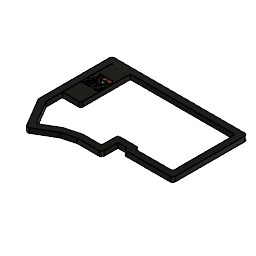
Right_top_cover (Autodesk Fusion 360 design; units mm, degrees)
part number: 2026-07-18-15-23-12-315
Autodesk Fusion 360 part; units mm, degrees
(part 1 of 2)
sketch "Right_enclosure_outline" plane through (0, 0, 0) normal (0, 0, 1) x (1, 0, 0)
  arc A0 (22.5, -32.5) -> (24.5, -34.5) centre (22.5, -34.5) cw
  line L0 (65.0462, 36) -> (-72.8538, 36)
  line L1 (0.5, -49.2983) -> (0.5, -34.5)
  line L2 (67.0462, -34.0424) -> (67.0462, 34)
  line L3 (-21.4538, -51.2983) -> (-1.5, -51.2983)
  line L4 (44.5449, -36.0424) -> (65.0462, -36.0424)
  line L5 (-39.1, -56.2) -> (-21.4538, -51.2983)
  line L6 (24.5, -34.5) -> (24.5, -36.0424)
  line L7 (2.5, -32.5) -> (22.5, -32.5)
  line L8 (-74.8538, 34) -> (-74.8538, 31.6376)
  arc A1 (0.5, -34.5) -> (2.5, -32.5) centre (2.5, -34.5) cw
  line L9 (-74.8538, 0.3904) -> (-74.8538, -39.752)
  line L10 (24.5, -36.0424) -> (44.5449, -36.0424)
  line L11 (-74.8538, 31.6376) -> (-74.8538, 0.3904)
  line L12 (-56.6719, -66.5254) -> (-39.1, -56.2)
  line L13 (-21.4538, -51.2983) -> (-1.5, -51.2983)
  line L14 (2.5, -32.5) -> (22.5, -32.5)
  line L15 (0.5, -49.2983) -> (0.5, -34.5)
  line L16 (24.5, -36.0424) -> (44.5449, -36.0424)
  arc A2 (-72.8538, 36) -> (-74.8538, 34) centre (-72.8538, 34) ccw
  line L17 (44.5449, -36.0424) -> (65.0462, -36.0424)
  line L18 (-74.8538, 0.3904) -> (-74.8538, -39.752)
  line L19 (67.0462, -34.0424) -> (67.0462, 34)
  line L20 (-74.8538, -39.752) -> (-59.4057, -65.8207)
  arc A3 (65.0462, -36.0424) -> (67.0462, -34.0424) centre (65.0462, -34.0424) ccw
  line L21 (-39.1, -56.2) -> (-21.4538, -51.2983)
  arc A4 (67.0462, 34) -> (65.0462, 36) centre (65.0462, 34) ccw
  arc A5 (-59.4057, -65.8207) -> (-56.6719, -66.5254) centre (-57.6851, -64.8011) ccw
  line L22 (24.5, -34.5) -> (24.5, -36.0424)
  arc A6 (-1.5, -51.2983) -> (0.5, -49.2983) centre (-1.5, -49.2983) ccw
  line L23 (-81.8538, 31.6376) -> (-81.8538, 0.3904)
  line L24 (-81.8538, 0.3904) -> (-81.8538, -41.6703)
  line L25 (-81.8538, -41.6703) -> (-62.3802, -74.532)
  line L26 (-58.2795, -75.5891) -> (-36.3436, -62.6994)
  arc A7 (17.5, -40.0424) -> (20.5, -43.0424) centre (20.5, -40.0424) ccw
  line L27 (-36.3436, -62.6994) -> (-20.4997, -58.2983)
  line L28 (71.0462, 43) -> (-78.8538, 43)
  line L29 (7.5, -55.2983) -> (7.5, -39.5)
  line L30 (20.5, -43.0424) -> (44.5449, -43.0424)
  line L31 (44.5449, -43.0424) -> (71.0462, -43.0424)
  line L32 (17.5, -39.5) -> (17.5, -40.0424)
  arc A8 (4.5, -58.2983) -> (7.5, -55.2983) centre (4.5, -55.2983) ccw
  line L33 (-81.8538, 40) -> (-81.8538, 31.6376)
  arc A9 (-62.3802, -74.532) -> (-58.2795, -75.5891) centre (-59.7994, -73.0026) ccw
  arc A10 (74.0462, 40) -> (71.0462, 43) centre (71.0462, 40) ccw
  arc A11 (-78.8538, 43) -> (-81.8538, 40) centre (-78.8538, 40) ccw
  line L34 (-20.4997, -58.2983) -> (4.5, -58.2983)
  line L35 (74.0462, -40.0424) -> (74.0462, 40)
  line L36 (7.5, -39.5) -> (17.5, -39.5)
  arc A12 (71.0462, -43.0424) -> (74.0462, -40.0424) centre (71.0462, -40.0424) ccw
  circle A13 centre (-78, 39) radius 1.6
  circle A14 centre (-60, -71) radius 1.6
  circle A15 centre (69.7169, -39.1925) radius 1.6
  circle A16 centre (69.6831, 39.8042) radius 1.6
  arc A17 (-1.5, -51.2983) -> (0.5, -49.2983) centre (-1.5, -49.2983) ccw
  arc A18 (2.5, -32.5) -> (0.5, -34.5) centre (2.5, -34.5) ccw
  arc A19 (24.5, -34.5) -> (22.5, -32.5) centre (22.5, -34.5) ccw
  arc A20 (65.0462, -36.0424) -> (67.0462, -34.0424) centre (65.0462, -34.0424) ccw
  arc A21 (67.0462, 34) -> (65.0462, 36) centre (65.0462, 34) ccw
  line L37 (-72.8247, 36.0109) -> (-54.3307, 36.0109)
  arc A22 (-72.8247, 36.0109) -> (-74.8247, 34.0109) centre (-72.8247, 34.0109) ccw
  line L38 (-72.8247, 36.0109) -> (-53.7017, 36.0109)
  line L39 (-53.7017, 36.0109) -> (-53.7017, -19.0891)
  line L40 (-55.7017, -21.0891) -> (-74.8247, -21.0891)
  line L41 (-74.8247, -21.0891) -> (-74.8247, 34.0109)
  arc A23 (-72.8247, 36.0109) -> (-74.8247, 34.0109) centre (-72.8247, 34.0109) ccw
  arc A24 (-55.7017, -21.0891) -> (-53.7017, -19.0891) centre (-55.7017, -19.0891) ccw
  point P0 (-74.8247, 36.0109)
  point P1 (-74.8247, 36.0109)
  dimension "d4" = 20.494
  dimension "d6" = 2
  dimension "d8" = 57.1
  dimension "d9" = 2
  constraint tangent L1 A17
  constraint tangent L3 A17
  constraint tangent L14 A18
  constraint tangent L15 A18
  constraint tangent L14 A19
  constraint tangent L22 A19
  constraint tangent L2 A20
  constraint tangent L4 A20
  constraint tangent L0 A21
  constraint tangent L2 A21
  constraint horizontal L37
  constraint coincident P1 L37
  constraint tangent L37 A22
  constraint perpendicular L38 L39
  constraint parallel L38 L40
  constraint parallel L39 L41
  constraint parallel L0 L38
  constraint coincident P1 P0
  constraint coincident P1 L38
  constraint coincident P1 L41
  constraint tangent L38 A23
  constraint tangent L41 A23
  constraint tangent L39 A24
  constraint tangent L40 A24
  constraint equal A23 A24
  measures "d4" distance of P1 L37.end
  measures "d6" radius of A22
  measures "d8" distance of P1 L40.end
  measures "d9" radius of A23
extrude "Extrude1" add sketch "Right_enclosure_outline" along normal blind 4.5 contours L0 A2 L37 A22 L38 L39 A23 | L23 L24 L25 L26 A7 L27 L28 L29 L30 L31 L32 A8 L33 A9 A10 A11 L34 L35 L36 A12 | A13 | A14 | A15 | A16 makes body 1
extrude "Extrude2" add sketch "Right_enclosure_outline" along normal blind 4.5 contours L0 A2 A22 L39 L40 L41 A23 A24 bodies 1
extrude "Extrude3" add 1 faces at (-67.7837, -2.0557, 4.5) along direction (0, 0, 1) blind 0.5 on bodies 1 bodies 1
extrude "Extrude4" add 1 faces at (-67.7837, -2.0557, 5) along direction (0, 0, 1) blind 0.5 on bodies 1 bodies 1
sketch "Sketch2" plane through (0, 0, 0) normal (0, 0, 1) x (1, 0, 0)
  circle A0 centre (-60, -71) radius 1.6
  circle A1 centre (-78, 39) radius 1.6
  circle A2 centre (69.6831, 39.8042) radius 1.6
  circle A3 centre (69.7169, -39.1925) radius 1.6
  circle A4 centre (-60, -71) radius 2.45
  circle A5 centre (-78, 39) radius 2.45
  circle A6 centre (69.6831, 39.8042) radius 2.45
  circle A7 centre (69.7169, -39.1925) radius 2.45
  dimension "d16" = 4.9
  dimension "d17" = 4.9
  dimension "d18" = 4.9
  dimension "d19" = 4.9
  constraint concentric A0 A4
  constraint concentric A1 A5
  constraint concentric A2 A6
  constraint concentric A3 A7
  measures "d16" diameter of A4
  measures "d17" diameter of A5
  measures "d18" diameter of A6
  measures "d19" diameter of A7
extrude "Extrude5" cut sketch "Sketch2" along normal blind 3.9 contours A0 | A1 | A2 | A3 | A4 | A5 | A6 | A7 bodies 1
sketch "Sketch3" plane through (0, 0, 0) normal (0, 0, -1) x (1, 0, 0)
  arc A0 (74.0462, 40.0424) -> (71.0462, 43.0424) centre (71.0462, 40.0424) ccw
  line L0 (71.0462, 43.0424) -> (20.5, 43.0424)
  arc A1 (20.5, 43.0424) -> (17.5, 40.0424) centre (20.5, 40.0424) ccw
  line L1 (17.5, 40.0424) -> (17.5, 39.5)
  line L2 (17.5, 39.5) -> (7.5, 39.5)
  line L3 (7.5, 39.5) -> (7.5, 55.2983)
  arc A2 (7.5, 55.2983) -> (4.5, 58.2983) centre (4.5, 55.2983) ccw
  line L4 (4.5, 58.2983) -> (-20.4997, 58.2983)
  line L5 (-20.4997, 58.2983) -> (-36.3436, 62.6994)
  line L6 (-36.3436, 62.6994) -> (-58.2795, 75.5891)
  arc A3 (-58.2795, 75.5891) -> (-62.3802, 74.532) centre (-59.7994, 73.0026) ccw
  line L7 (-62.3802, 74.532) -> (-81.8538, 41.6703)
  line L8 (-81.8538, 41.6703) -> (-81.8538, -40)
  arc A4 (-81.8538, -40) -> (-78.8538, -43) centre (-78.8538, -40) ccw
  line L9 (-78.8538, -43) -> (71.0462, -43)
  arc A5 (71.0462, -43) -> (74.0462, -40) centre (71.0462, -40) ccw
  line L10 (74.0462, -40) -> (74.0462, 40.0424)
  line L11 (24.5, 34.5) -> (24.5, 36.0424)
  line L12 (24.5, 36.0424) -> (65.0462, 36.0424)
  arc A6 (67.0462, 34.0424) -> (65.0462, 36.0424) centre (65.0462, 34.0424) ccw
  line L13 (67.0462, 34.0424) -> (67.0462, -34)
  arc A7 (65.0462, -36) -> (67.0462, -34) centre (65.0462, -34) ccw
  line L14 (65.0462, -36) -> (-53.7017, -36)
  line L15 (-53.7017, -36) -> (-53.7017, 19.0891)
  arc A8 (-53.7017, 19.0891) -> (-55.7017, 21.0891) centre (-55.7017, 19.0891) ccw
  line L16 (-55.7017, 21.0891) -> (-74.8247, 21.0891)
  line L17 (-74.8247, 21.0891) -> (-74.8247, -34.0109)
  arc A9 (-74.8247, -34.0109) -> (-73.5427, -35.8776) centre (-72.8247, -34.0109) ccw
  arc A10 (-74.8538, -34) -> (-73.5427, -35.8776) centre (-72.8538, -34) ccw
  line L18 (-74.8538, -34) -> (-74.8538, 39.752)
  line L19 (-74.8538, 39.752) -> (-59.4057, 65.8207)
  arc A11 (-56.6719, 66.5254) -> (-59.4057, 65.8207) centre (-57.6851, 64.8011) ccw
  line L20 (-56.6719, 66.5254) -> (-39.1, 56.2)
  line L21 (-39.1, 56.2) -> (-21.4538, 51.2983)
  line L22 (-21.4538, 51.2983) -> (-1.5, 51.2983)
  arc A12 (0.5, 49.2983) -> (-1.5, 51.2983) centre (-1.5, 49.2983) ccw
  line L23 (0.5, 49.2983) -> (0.5, 34.5)
  arc A13 (0.5, 34.5) -> (2.5, 32.5) centre (2.5, 34.5) ccw
  line L24 (2.5, 32.5) -> (22.5, 32.5)
  arc A14 (22.5, 32.5) -> (24.5, 34.5) centre (22.5, 34.5) ccw
  circle A15 centre (69.7169, 39.1925) radius 2.45
  circle A16 centre (-60, 71) radius 2.45
  circle A17 centre (69.6831, -39.8042) radius 2.45
  circle A18 centre (-78, -39) radius 2.45
  line L25 (-74, 19) -> (-55, 19)
  line L26 (-55, 19) -> (-55, -33)
  line L27 (-55, -33) -> (-74, -33)
  line L28 (-74, -33) -> (-74, 19)
  constraint perpendicular L25 L26
  constraint parallel L25 L27
  constraint parallel L26 L28
  constraint perpendicular L15 L25
extrude "Extrude6" cut sketch "Sketch3" against normal blind 4.5 contours L25 L26 L27 L28 bodies 1
sketch "Sketch4" plane through (0, 0, 5.5) normal (0, 0, 1) x (-1, 0, 0)
  line L0 (-24.5, 36.0424) -> (-24.5, 34.5)
  arc A0 (-24.5, 34.5) -> (-22.5, 32.5) centre (-22.5, 34.5) ccw
  line L1 (-22.5, 32.5) -> (-2.5, 32.5)
  arc A1 (-2.5, 32.5) -> (-0.5, 34.5) centre (-2.5, 34.5) ccw
  line L2 (-0.5, 34.5) -> (-0.5, 49.2983)
  arc A2 (1.5, 51.2983) -> (-0.5, 49.2983) centre (1.5, 49.2983) ccw
  line L3 (1.5, 51.2983) -> (21.4538, 51.2983)
  line L4 (21.4538, 51.2983) -> (39.1, 56.2)
  line L5 (39.1, 56.2) -> (56.6719, 66.5254)
  arc A3 (59.4057, 65.8207) -> (56.6719, 66.5254) centre (57.6851, 64.8011) ccw
  line L6 (59.4057, 65.8207) -> (74.8538, 39.752)
  line L7 (74.8538, 39.752) -> (74.8538, -34)
  arc A4 (73.5427, -35.8776) -> (74.8538, -34) centre (72.8538, -34) ccw
  arc A5 (73.5427, -35.8776) -> (74.8247, -34.0109) centre (72.8247, -34.0109) ccw
  line L8 (74.8247, -34.0109) -> (74.8247, 21.0891)
  line L9 (74.8247, 21.0891) -> (55.7017, 21.0891)
  arc A6 (55.7017, 21.0891) -> (53.7017, 19.0891) centre (55.7017, 19.0891) ccw
  line L10 (53.7017, 19.0891) -> (53.7017, -36)
  line L11 (53.7017, -36) -> (-65.0462, -36)
  arc A7 (-67.0462, -34) -> (-65.0462, -36) centre (-65.0462, -34) ccw
  line L12 (-67.0462, -34) -> (-67.0462, 34.0424)
  arc A8 (-65.0462, 36.0424) -> (-67.0462, 34.0424) centre (-65.0462, 34.0424) ccw
  line L13 (-65.0462, 36.0424) -> (-24.5, 36.0424)
  arc A9 (-71.0462, 43.0424) -> (-74.0462, 40.0424) centre (-71.0462, 40.0424) ccw
  line L14 (-74.0462, 40.0424) -> (-74.0462, -40)
  arc A10 (-74.0462, -40) -> (-71.0462, -43) centre (-71.0462, -40) ccw
  line L15 (-71.0462, -43) -> (78.8538, -43)
  arc A11 (78.8538, -43) -> (81.8538, -40) centre (78.8538, -40) ccw
  line L16 (81.8538, -40) -> (81.8538, 41.6703)
  line L17 (81.8538, 41.6703) -> (62.3802, 74.532)
  arc A12 (62.3802, 74.532) -> (58.2795, 75.5891) centre (59.7994, 73.0026) ccw
  line L18 (58.2795, 75.5891) -> (36.3436, 62.6994)
  line L19 (36.3436, 62.6994) -> (20.4997, 58.2983)
  line L20 (20.4997, 58.2983) -> (-4.5, 58.2983)
  arc A13 (-4.5, 58.2983) -> (-7.5, 55.2983) centre (-4.5, 55.2983) ccw
  line L21 (-7.5, 55.2983) -> (-7.5, 39.5)
  line L22 (-7.5, 39.5) -> (-17.5, 39.5)
  line L23 (-17.5, 39.5) -> (-17.5, 40.0424)
  arc A14 (-17.5, 40.0424) -> (-20.5, 43.0424) centre (-20.5, 40.0424) ccw
  line L24 (-20.5, 43.0424) -> (-71.0462, 43.0424)
  spline S0 degree 3 poles (70.819, -18.6802) (70.9391, -18.6554) (71.1029, -18.5716) (71.16, -18.503) knots 0 0 0 0 1 1 1 1
  spline S1 degree 3 poles (71.16, -18.503) (71.2553, -18.3906) (71.2896, -18.2859) (71.2896, -18.1087) knots 0 0 0 0 1 1 1 1
  spline S2 degree 3 poles (71.2896, -18.1087) (71.2877, -17.9106) (71.2439, -17.8039) (71.1105, -17.6839) knots 0 0 0 0 1 1 1 1
  spline S3 degree 3 poles (71.1105, -17.6839) (70.9486, -17.5391) (70.7562, -17.5086) (70.379, -17.5677) knots 0 0 0 0 1 1 1 1
  spline S4 degree 3 poles (70.379, -17.5677) (70.1466, -17.6058) (69.9866, -17.5963) (69.9142, -17.5448) knots 0 0 0 0 1 1 1 1
  spline S5 degree 3 poles (69.9142, -17.5448) (69.8399, -17.4896) (69.7465, -17.3429) (69.718, -17.2381) knots 0 0 0 0 1 1 1 1
  spline S6 degree 3 poles (69.718, -17.2381) (69.6856, -17.1181) (69.6703, -11.8108) (69.7008, -11.6031) knots 0 0 0 0 1 1 1 1
  spline S7 degree 3 poles (69.7008, -11.6031) (69.7122, -11.5307) (69.7465, -11.4164) (69.7789, -11.3517) knots 0 0 0 0 1 1 1 1
  spline S8 degree 3 poles (69.7789, -11.3517) (69.8246, -11.2564) (69.8551, -11.2221) (69.9256, -11.1802) knots 0 0 0 0 1 1 1 1
  spline S9 degree 3 poles (69.9256, -11.1802) (70.0285, -11.1193) (70.1256, -11.1155) (70.4819, -11.1536) knots 0 0 0 0 1 1 1 1
  spline S10 degree 3 poles (70.4819, -11.1536) (70.9372, -11.2031) (71.1315, -11.1345) (71.2458, -10.8792) knots 0 0 0 0 1 1 1 1
  spline S11 degree 3 poles (71.2458, -10.8792) (71.2801, -10.8049) (71.2896, -10.7478) (71.2896, -10.6202) knots 0 0 0 0 1 1 1 1
  spline S12 degree 3 poles (71.2896, -10.6202) (71.2896, -10.4716) (71.2839, -10.4449) (71.2248, -10.3249) knots 0 0 0 0 1 1 1 1
  spline S13 degree 3 poles (71.2248, -10.3249) (71.0705, -10.0201) (70.7733, -9.9534) (70.0628, -10.0677) knots 0 0 0 0 1 1 1 1
  spline S14 degree 3 poles (70.0628, -10.0677) (69.5675, -10.1458) (69.2855, -10.1687) (68.8626, -10.1687) knots 0 0 0 0 1 1 1 1
  spline S15 degree 3 poles (68.8626, -10.1687) (68.5083, -10.1668) (68.4454, -10.161) (67.7577, -10.0506) knots 0 0 0 0 1 1 1 1
  spline S16 degree 3 poles (67.7577, -10.0506) (67.3558, -9.9877) (67.0929, -10.0067) (66.8967, -10.1172) knots 0 0 0 0 1 1 1 1
  spline S17 degree 3 poles (66.8967, -10.1172) (66.7233, -10.2144) (66.6547, -10.3401) (66.6395, -10.584) knots 0 0 0 0 1 1 1 1
  spline S18 degree 3 poles (66.6395, -10.584) (66.6242, -10.8526) (66.7138, -11.0297) (66.9195, -11.125) knots 0 0 0 0 1 1 1 1
  spline S19 degree 3 poles (66.9195, -11.125) (66.99, -11.1574) (67.0414, -11.165) (67.2148, -11.165) knots 0 0 0 0 1 1 1 1
  spline S20 degree 3 poles (67.2148, -11.165) (67.3291, -11.165) (67.5158, -11.1536) (67.6282, -11.1402) knots 0 0 0 0 1 1 1 1
  spline S21 degree 3 poles (67.6282, -11.1402) (67.8796, -11.1097) (67.9635, -11.1269) (68.0644, -11.2278) knots 0 0 0 0 1 1 1 1
  spline S22 degree 3 poles (68.0644, -11.2278) (68.1025, -11.2679) (68.154, -11.3498) (68.1787, -11.4126) knots 0 0 0 0 1 1 1 1
  line L25 (68.1787, -11.4126) -> (68.2244, -11.5269)
  line L26 (68.2244, -11.5269) -> (68.2244, -14.3463)
  spline S23 degree 3 poles (68.2244, -14.3463) (68.2244, -17.0267) (68.2225, -17.1714) (68.1901, -17.2743) knots 0 0 0 0 1 1 1 1
  spline S24 degree 3 poles (68.1901, -17.2743) (68.0949, -17.5696) (67.9501, -17.6363) (67.5482, -17.5658) knots 0 0 0 0 1 1 1 1
  spline S25 degree 3 poles (67.5482, -17.5658) (67.1786, -17.501) (66.969, -17.5429) (66.7957, -17.7163) knots 0 0 0 0 1 1 1 1
  spline S26 degree 3 poles (66.7957, -17.7163) (66.6814, -17.8287) (66.6338, -17.9468) (66.6338, -18.1106) knots 0 0 0 0 1 1 1 1
  spline S27 degree 3 poles (66.6338, -18.1106) (66.6338, -18.2744) (66.6852, -18.4078) (66.7862, -18.5107) knots 0 0 0 0 1 1 1 1
  spline S28 degree 3 poles (66.7862, -18.5107) (66.9805, -18.7069) (67.2567, -18.7393) (67.9101, -18.644) knots 0 0 0 0 1 1 1 1
  spline S29 degree 3 poles (67.9101, -18.644) (68.7655, -18.5221) (69.1807, -18.5221) (70.0056, -18.6421) knots 0 0 0 0 1 1 1 1
  spline S30 degree 3 poles (70.0056, -18.6421) (70.3942, -18.6993) (70.659, -18.7107) (70.819, -18.6802) knots 0 0 0 0 1 1 1 1
  spline S31 degree 3 poles (63.0143, -18.5926) (63.3648, -18.5392) (63.7648, -18.404) (64.062, -18.2382) knots 0 0 0 0 1 1 1 1
  spline S32 degree 3 poles (64.062, -18.2382) (64.2582, -18.1297) (64.5592, -17.8953) (64.6983, -17.7449) knots 0 0 0 0 1 1 1 1
  spline S33 degree 3 poles (64.6983, -17.7449) (65.045, -17.3696) (65.3612, -16.7123) (65.445, -16.1923) knots 0 0 0 0 1 1 1 1
  spline S34 degree 3 poles (65.445, -16.1923) (65.5098, -15.7922) (65.4984, -15.0055) (65.426, -14.7026) knots 0 0 0 0 1 1 1 1
  spline S35 degree 3 poles (65.426, -14.7026) (65.3326, -14.3159) (65.1155, -13.7939) (64.8774, -13.3748) knots 0 0 0 0 1 1 1 1
  spline S36 degree 3 poles (64.8774, -13.3748) (64.5802, -12.8566) (64.1268, -12.2718) (63.6448, -11.7879) knots 0 0 0 0 1 1 1 1
  spline S37 degree 3 poles (63.6448, -11.7879) (62.9343, -11.0735) (62.0884, -10.4506) (60.9664, -9.8181) knots 0 0 0 0 1 1 1 1
  spline S38 degree 3 poles (60.9664, -9.8181) (60.8826, -9.7705) (60.7797, -9.7115) (60.7378, -9.6886) knots 0 0 0 0 1 1 1 1
  spline S39 degree 3 poles (60.7378, -9.6886) (60.5911, -9.6048) (60.3663, -9.4981) (60.3377, -9.4981) knots 0 0 0 0 1 1 1 1
  spline S40 degree 3 poles (60.3377, -9.4981) (60.2577, -9.4981) (59.791, -9.7762) (59.0614, -10.2601) knots 0 0 0 0 1 1 1 1
  spline S41 degree 3 poles (59.0614, -10.2601) (58.6556, -10.5287) (58.2289, -10.843) (57.9851, -11.0507) knots 0 0 0 0 1 1 1 1
  spline S42 degree 3 poles (57.9851, -11.0507) (57.9584, -11.0735) (57.8689, -11.1516) (57.785, -11.224) knots 0 0 0 0 1 1 1 1
  spline S43 degree 3 poles (57.785, -11.224) (57.1011, -11.8089) (56.282, -12.7252) (55.9086, -13.3253) knots 0 0 0 0 1 1 1 1
  spline S44 degree 3 poles (55.9086, -13.3253) (55.3562, -14.2149) (55.1371, -15.3331) (55.3295, -16.2799) knots 0 0 0 0 1 1 1 1
  spline S45 degree 3 poles (55.3295, -16.2799) (55.4628, -16.9276) (55.8858, -17.6248) (56.3715, -18.0001) knots 0 0 0 0 1 1 1 1
  spline S46 degree 3 poles (56.3715, -18.0001) (57.0173, -18.4992) (57.8631, -18.705) (58.6232, -18.5488) knots 0 0 0 0 1 1 1 1
  spline S47 degree 3 poles (58.6232, -18.5488) (58.9185, -18.4878) (59.1452, -18.383) (59.5186, -18.1354) knots 0 0 0 0 1 1 1 1
  spline S48 degree 3 poles (59.5186, -18.1354) (59.8081, -17.943) (59.9586, -17.8191) (60.2177, -17.5639) knots 0 0 0 0 1 1 1 1
  spline S49 degree 3 poles (60.2177, -17.5639) (60.3396, -17.442) (60.452, -17.3467) (60.4654, -17.3505) knots 0 0 0 0 1 1 1 1
  spline S50 degree 3 poles (60.4654, -17.3505) (60.4806, -17.3524) (60.5568, -17.4286) (60.6349, -17.5182) knots 0 0 0 0 1 1 1 1
  spline S51 degree 3 poles (60.6349, -17.5182) (60.854, -17.7715) (61.1455, -18.0497) (61.3131, -18.1716) knots 0 0 0 0 1 1 1 1
  spline S52 degree 3 poles (61.3131, -18.1716) (61.8389, -18.5469) (62.3951, -18.684) (63.0143, -18.5926) knots 0 0 0 0 1 1 1 1
  spline S53 degree 3 poles (60.7206, -16.0018) (60.7016, -15.9942) (60.6902, -15.9675) (60.6902, -15.9275) knots 0 0 0 0 1 1 1 1
  spline S54 degree 3 poles (60.6902, -15.9275) (60.6902, -15.8913) (60.6806, -15.857) (60.6711, -15.8513) knots 0 0 0 0 1 1 1 1
  spline S55 degree 3 poles (60.6711, -15.8513) (60.6463, -15.836) (60.6463, -15.7275) (60.6711, -15.7275) knots 0 0 0 0 1 1 1 1
  spline S56 degree 3 poles (60.6711, -15.7275) (60.6959, -15.7275) (60.6806, -15.5732) (60.6387, -15.4093) knots 0 0 0 0 1 1 1 1
  spline S57 degree 3 poles (60.6387, -15.4093) (60.6159, -15.316) (60.6006, -15.2893) (60.574, -15.2893) knots 0 0 0 0 1 1 1 1
  spline S58 degree 3 poles (60.574, -15.2893) (60.532, -15.2893) (60.5282, -15.3103) (60.5606, -15.3426) knots 0 0 0 0 1 1 1 1
  spline S59 degree 3 poles (60.5606, -15.3426) (60.5778, -15.3598) (60.5778, -15.3655) (60.5625, -15.3655) knots 0 0 0 0 1 1 1 1
  spline S60 degree 3 poles (60.5625, -15.3655) (60.5492, -15.3655) (60.534, -15.3579) (60.5282, -15.3465) knots 0 0 0 0 1 1 1 1
  spline S61 degree 3 poles (60.5282, -15.3465) (60.5073, -15.3141) (60.4616, -15.3255) (60.4616, -15.3636) knots 0 0 0 0 1 1 1 1
  spline S62 degree 3 poles (60.4616, -15.3636) (60.4616, -15.4227) (60.4254, -15.4303) (60.4025, -15.3769) knots 0 0 0 0 1 1 1 1
  spline S63 degree 3 poles (60.4025, -15.3769) (60.3835, -15.3388) (60.3739, -15.3331) (60.3377, -15.3465) knots 0 0 0 0 1 1 1 1
  spline S64 degree 3 poles (60.3377, -15.3465) (60.3015, -15.3598) (60.2958, -15.3579) (60.3034, -15.3255) knots 0 0 0 0 1 1 1 1
  spline S65 degree 3 poles (60.3034, -15.3255) (60.3111, -15.3007) (60.3034, -15.2893) (60.2844, -15.2893) knots 0 0 0 0 1 1 1 1
  spline S66 degree 3 poles (60.2844, -15.2893) (60.2615, -15.2893) (60.2558, -15.276) (60.2634, -15.2283) knots 0 0 0 0 1 1 1 1
  spline S67 degree 3 poles (60.2634, -15.2283) (60.2901, -15.0645) (60.2825, -15.0169) (60.2196, -14.9426) knots 0 0 0 0 1 1 1 1
  spline S68 degree 3 poles (60.2196, -14.9426) (60.1872, -14.9026) (60.1549, -14.8454) (60.1472, -14.815) knots 0 0 0 0 1 1 1 1
  spline S69 degree 3 poles (60.1472, -14.815) (60.1415, -14.7845) (60.1225, -14.7483) (60.1053, -14.735) knots 0 0 0 0 1 1 1 1
  spline S70 degree 3 poles (60.1053, -14.735) (60.0825, -14.714) (60.0729, -14.7159) (60.052, -14.7426) knots 0 0 0 0 1 1 1 1
  spline S71 degree 3 poles (60.052, -14.7426) (60.0234, -14.7826) (59.9986, -14.7826) (59.9263, -14.7464) knots 0 0 0 0 1 1 1 1
  spline S72 degree 3 poles (59.9263, -14.7464) (59.8729, -14.7178) (59.871, -14.7102) (59.8767, -14.6264) knots 0 0 0 0 1 1 1 1
  spline S73 degree 3 poles (59.8767, -14.6264) (59.8843, -14.5292) (59.9072, -14.4721) (59.9548, -14.4321) knots 0 0 0 0 1 1 1 1
  spline S74 degree 3 poles (59.9548, -14.4321) (59.972, -14.4187) (59.9853, -14.3825) (59.9853, -14.352) knots 0 0 0 0 1 1 1 1
  spline S75 degree 3 poles (59.9853, -14.352) (59.9853, -14.3178) (60.0025, -14.2797) (60.0329, -14.253) knots 0 0 0 0 1 1 1 1
  spline S76 degree 3 poles (60.0329, -14.253) (60.0748, -14.213) (60.0787, -14.2016) (60.0672, -14.0777) knots 0 0 0 0 1 1 1 1
  spline S77 degree 3 poles (60.0672, -14.0777) (60.0615, -14.0053) (60.0672, -13.8415) (60.0787, -13.712) knots 0 0 0 0 1 1 1 1
  spline S78 degree 3 poles (60.0787, -13.712) (60.1053, -13.4472) (60.0958, -13.3748) (60.0387, -13.3595) knots 0 0 0 0 1 1 1 1
  spline S79 degree 3 poles (60.0387, -13.3595) (60.0082, -13.35) (60.0025, -13.3367) (60.0082, -13.3005) knots 0 0 0 0 1 1 1 1
  spline S80 degree 3 poles (60.0082, -13.3005) (60.0177, -13.2567) (60.012, -13.2529) (59.9301, -13.2471) knots 0 0 0 0 1 1 1 1
  line L27 (59.9301, -13.2471) -> (59.8424, -13.2414)
  line L28 (59.8424, -13.2414) -> (59.8367, -13.1614)
  spline S81 degree 3 poles (59.8367, -13.1614) (59.8329, -13.1119) (59.8386, -13.0795) (59.852, -13.0795) knots 0 0 0 0 1 1 1 1
  spline S82 degree 3 poles (59.852, -13.0795) (59.8824, -13.0795) (59.8691, -12.428) (59.8367, -12.4166) knots 0 0 0 0 1 1 1 1
  spline S83 degree 3 poles (59.8367, -12.4166) (59.8196, -12.4109) (59.8139, -12.4909) (59.8139, -12.7709) knots 0 0 0 0 1 1 1 1
  spline S84 degree 3 poles (59.8139, -12.7709) (59.8139, -13.1176) (59.812, -13.1348) (59.7758, -13.1462) knots 0 0 0 0 1 1 1 1
  spline S85 degree 3 poles (59.7758, -13.1462) (59.7396, -13.1576) (59.7377, -13.1748) (59.7377, -13.6682) knots 0 0 0 0 1 1 1 1
  line L29 (59.7377, -13.6682) -> (59.7377, -14.1787)
  line L30 (59.7377, -14.1787) -> (59.551, -14.192)
  spline S86 degree 3 poles (59.551, -14.192) (59.45, -14.1977) (59.3071, -14.2092) (59.2366, -14.2149) knots 0 0 0 0 1 1 1 1
  spline S87 degree 3 poles (59.2366, -14.2149) (59.1604, -14.2225) (59.0881, -14.2187) (59.0652, -14.2073) knots 0 0 0 0 1 1 1 1
  spline S88 degree 3 poles (59.0652, -14.2073) (59.0423, -14.1958) (59.008, -14.1825) (58.989, -14.1768) knots 0 0 0 0 1 1 1 1
  spline S89 degree 3 poles (58.989, -14.1768) (58.9661, -14.1692) (58.9566, -14.1463) (58.9566, -14.1006) knots 0 0 0 0 1 1 1 1
  spline S90 degree 3 poles (58.9566, -14.1006) (58.9566, -14.0434) (58.9509, -14.0339) (58.9033, -14.0282) knots 0 0 0 0 1 1 1 1
  line L31 (58.9033, -14.0282) -> (58.8518, -14.0225)
  line L32 (58.8518, -14.0225) -> (58.8385, -13.7367)
  spline S91 degree 3 poles (58.8385, -13.7367) (58.8214, -13.3329) (58.808, -13.2567) (58.7642, -13.2452) knots 0 0 0 0 1 1 1 1
  spline S92 degree 3 poles (58.7642, -13.2452) (58.7337, -13.2376) (58.728, -13.2186) (58.728, -13.1367) knots 0 0 0 0 1 1 1 1
  line L33 (58.728, -13.1367) -> (58.728, -13.0376)
  line L34 (58.728, -13.0376) -> (58.6709, -13.0509)
  spline S93 degree 3 poles (58.6709, -13.0509) (58.6385, -13.0586) (58.5661, -13.0643) (58.5089, -13.0643) knots 0 0 0 0 1 1 1 1
  line L35 (58.5089, -13.0643) -> (58.4042, -13.0662)
  line L36 (58.4042, -13.0662) -> (58.4042, -13.6243)
  line L37 (58.4042, -13.6243) -> (58.4042, -14.1844)
  line L38 (58.4042, -14.1844) -> (58.3032, -14.1863)
  spline S94 degree 3 poles (58.3032, -14.1863) (58.2499, -14.1863) (58.1089, -14.1882) (57.9908, -14.1882) knots 0 0 0 0 1 1 1 1
  line L39 (57.9908, -14.1882) -> (57.7774, -14.1901)
  line L40 (57.7774, -14.1901) -> (57.7717, -14.2397)
  spline S95 degree 3 poles (57.7717, -14.2397) (57.7679, -14.2682) (57.7546, -14.2892) (57.7374, -14.2892) knots 0 0 0 0 1 1 1 1
  spline S96 degree 3 poles (57.7374, -14.2892) (57.7165, -14.2892) (57.7069, -14.2587) (57.6974, -14.1749) knots 0 0 0 0 1 1 1 1
  spline S97 degree 3 poles (57.6974, -14.1749) (57.6917, -14.112) (57.6669, -14.0053) (57.6422, -13.9368) knots 0 0 0 0 1 1 1 1
  spline S98 degree 3 poles (57.6422, -13.9368) (57.6174, -13.8682) (57.5926, -13.7463) (57.5869, -13.6605) knots 0 0 0 0 1 1 1 1
  line L41 (57.5869, -13.6605) -> (57.5755, -13.5081)
  line L42 (57.5755, -13.5081) -> (57.4707, -13.5024)
  spline S99 degree 3 poles (57.4707, -13.5024) (57.4136, -13.4986) (57.3602, -13.4853) (57.3526, -13.4738) knots 0 0 0 0 1 1 1 1
  spline S100 degree 3 poles (57.3526, -13.4738) (57.345, -13.4605) (57.3374, -13.3195) (57.3374, -13.1576) knots 0 0 0 0 1 1 1 1
  spline S101 degree 3 poles (57.3374, -13.1576) (57.3374, -12.9004) (57.3336, -12.8681) (57.3069, -12.8776) knots 0 0 0 0 1 1 1 1
  spline S102 degree 3 poles (57.3069, -12.8776) (57.2897, -12.8833) (57.2516, -12.889) (57.2231, -12.889) knots 0 0 0 0 1 1 1 1
  spline S103 degree 3 poles (57.2231, -12.889) (57.1716, -12.889) (57.1678, -12.8947) (57.1621, -12.9709) knots 0 0 0 0 1 1 1 1
  line L43 (57.1621, -12.9709) -> (57.1564, -13.0509)
  line L44 (57.1564, -13.0509) -> (56.9887, -13.0509)
  line L45 (56.9887, -13.0509) -> (56.823, -13.0509)
  line L46 (56.823, -13.0509) -> (56.823, -13.4186)
  spline S104 degree 3 poles (56.823, -13.4186) (56.823, -13.6434) (56.8154, -13.8015) (56.8021, -13.8244) knots 0 0 0 0 1 1 1 1
  spline S105 degree 3 poles (56.8021, -13.8244) (56.7906, -13.8453) (56.724, -13.9006) (56.6535, -13.9463) knots 0 0 0 0 1 1 1 1
  spline S106 degree 3 poles (56.6535, -13.9463) (56.5373, -14.0206) (56.522, -14.0396) (56.4934, -14.1292) knots 0 0 0 0 1 1 1 1
  spline S107 degree 3 poles (56.4934, -14.1292) (56.4763, -14.1825) (56.4592, -14.2492) (56.4592, -14.2778) knots 0 0 0 0 1 1 1 1
  spline S108 degree 3 poles (56.4592, -14.2778) (56.4573, -14.3082) (56.4496, -14.2911) (56.4344, -14.2282) knots 0 0 0 0 1 1 1 1
  spline S109 degree 3 poles (56.4344, -14.2282) (56.423, -14.1749) (56.4077, -14.1234) (56.3982, -14.1158) knots 0 0 0 0 1 1 1 1
  spline S110 degree 3 poles (56.3982, -14.1158) (56.3906, -14.1082) (56.3849, -14.0777) (56.3849, -14.0492) knots 0 0 0 0 1 1 1 1
  spline S111 degree 3 poles (56.3849, -14.0492) (56.3849, -14.0206) (56.3772, -13.992) (56.3677, -13.9863) knots 0 0 0 0 1 1 1 1
  spline S112 degree 3 poles (56.3677, -13.9863) (56.3468, -13.973) (56.3277, -13.8587) (56.3163, -13.6662) knots 0 0 0 0 1 1 1 1
  spline S113 degree 3 poles (56.3163, -13.6662) (56.3087, -13.55) (56.2991, -13.5177) (56.2763, -13.5177) knots 0 0 0 0 1 1 1 1
  spline S114 degree 3 poles (56.2763, -13.5177) (56.261, -13.5177) (56.2439, -13.5005) (56.2382, -13.4796) knots 0 0 0 0 1 1 1 1
  spline S115 degree 3 poles (56.2382, -13.4796) (56.2325, -13.4586) (56.2153, -13.4415) (56.202, -13.4415) knots 0 0 0 0 1 1 1 1
  spline S116 degree 3 poles (56.202, -13.4415) (56.1601, -13.4415) (56.1696, -13.4129) (56.2629, -13.2757) knots 0 0 0 0 1 1 1 1
  spline S117 degree 3 poles (56.2629, -13.2757) (56.4934, -12.9404) (56.9316, -12.4242) (57.3393, -12.0127) knots 0 0 0 0 1 1 1 1
  spline S118 degree 3 poles (57.3393, -12.0127) (58.0384, -11.306) (58.6823, -10.8049) (59.7472, -10.1325) knots 0 0 0 0 1 1 1 1
  spline S119 degree 3 poles (59.7472, -10.1325) (59.9758, -9.9877) (60.2768, -9.8105) (60.3168, -9.7972) knots 0 0 0 0 1 1 1 1
  spline S120 degree 3 poles (60.3168, -9.7972) (60.353, -9.782) (60.5111, -9.862) (60.8673, -10.0734) knots 0 0 0 0 1 1 1 1
  spline S121 degree 3 poles (60.8673, -10.0734) (60.9721, -10.1344) (61.0578, -10.1839) (61.0616, -10.1839) knots 0 0 0 0 1 1 1 1
  spline S122 degree 3 poles (61.0616, -10.1839) (61.0788, -10.1839) (61.6446, -10.5344) (61.8617, -10.6792) knots 0 0 0 0 1 1 1 1
  spline S123 degree 3 poles (61.8617, -10.6792) (62.9952, -11.4336) (63.9306, -12.3537) (64.5192, -13.2929) knots 0 0 0 0 1 1 1 1
  spline S124 degree 3 poles (64.5192, -13.2929) (64.563, -13.3653) (64.5954, -13.4319) (64.5916, -13.4453) knots 0 0 0 0 1 1 1 1
  spline S125 degree 3 poles (64.5916, -13.4453) (64.5859, -13.4605) (64.5535, -13.4662) (64.504, -13.4643) knots 0 0 0 0 1 1 1 1
  line L47 (64.504, -13.4643) -> (64.4259, -13.4586)
  line L48 (64.4259, -13.4586) -> (64.4202, -13.7024)
  line L49 (64.4202, -13.7024) -> (64.4144, -13.9463)
  line L50 (64.4144, -13.9463) -> (64.2239, -13.9463)
  line L51 (64.2239, -13.9463) -> (64.0334, -13.9463)
  line L52 (64.0334, -13.9463) -> (64.0277, -13.7615)
  line L53 (64.0277, -13.7615) -> (64.022, -13.5748)
  line L54 (64.022, -13.5748) -> (63.8429, -13.5748)
  line L55 (63.8429, -13.5748) -> (63.662, -13.5748)
  line L56 (63.662, -13.5748) -> (63.662, -13.4434)
  line L57 (63.662, -13.4434) -> (63.662, -13.31)
  line L58 (63.662, -13.31) -> (63.561, -13.3043)
  line L59 (63.561, -13.3043) -> (63.4619, -13.2986)
  line L60 (63.4619, -13.2986) -> (63.4562, -13.0852)
  spline S126 degree 3 poles (63.4562, -13.0852) (63.4524, -12.9195) (63.4448, -12.8719) (63.4238, -12.8623) knots 0 0 0 0 1 1 1 1
  spline S127 degree 3 poles (63.4238, -12.8623) (63.3991, -12.8528) (63.3953, -12.9157) (63.3953, -13.3176) knots 0 0 0 0 1 1 1 1
  line L61 (63.3953, -13.3176) -> (63.3953, -13.7844)
  line L62 (63.3953, -13.7844) -> (63.2448, -13.7844)
  spline S128 degree 3 poles (63.2448, -13.7844) (63.1248, -13.7844) (63.0924, -13.7786) (63.0828, -13.7539) knots 0 0 0 0 1 1 1 1
  spline S129 degree 3 poles (63.0828, -13.7539) (63.0771, -13.7367) (63.0714, -13.6224) (63.0714, -13.4967) knots 0 0 0 0 1 1 1 1
  line L63 (63.0714, -13.4967) -> (63.0714, -13.27)
  line L64 (63.0714, -13.27) -> (62.9857, -13.27)
  spline S130 degree 3 poles (62.9857, -13.27) (62.9076, -13.27) (62.9, -13.2662) (62.9, -13.2224) knots 0 0 0 0 1 1 1 1
  spline S131 degree 3 poles (62.9, -13.2224) (62.9, -13.1957) (62.8904, -13.1748) (62.8809, -13.1748) knots 0 0 0 0 1 1 1 1
  spline S132 degree 3 poles (62.8809, -13.1748) (62.8695, -13.1748) (62.8619, -13.2357) (62.8619, -13.3176) knots 0 0 0 0 1 1 1 1
  line L65 (62.8619, -13.3176) -> (62.8619, -13.4624)
  line L66 (62.8619, -13.4624) -> (62.7418, -13.4567)
  line L67 (62.7418, -13.4567) -> (62.6237, -13.451)
  line L68 (62.6237, -13.451) -> (62.618, -13.1309)
  spline S133 degree 3 poles (62.618, -13.1309) (62.6142, -12.8871) (62.6085, -12.8109) (62.5894, -12.8185) knots 0 0 0 0 1 1 1 1
  spline S134 degree 3 poles (62.5894, -12.8185) (62.5723, -12.8242) (62.5647, -12.9157) (62.5609, -13.15) knots 0 0 0 0 1 1 1 1
  spline S135 degree 3 poles (62.5609, -13.15) (62.5571, -13.4129) (62.5513, -13.4796) (62.5266, -13.4986) knots 0 0 0 0 1 1 1 1
  spline S136 degree 3 poles (62.5266, -13.4986) (62.4847, -13.5348) (62.0122, -13.5691) (61.9646, -13.5405) knots 0 0 0 0 1 1 1 1
  spline S137 degree 3 poles (61.9646, -13.5405) (61.9456, -13.5272) (61.9113, -13.5177) (61.8903, -13.5177) knots 0 0 0 0 1 1 1 1
  spline S138 degree 3 poles (61.8903, -13.5177) (61.8579, -13.5177) (61.8522, -13.531) (61.8522, -13.6129) knots 0 0 0 0 1 1 1 1
  spline S139 degree 3 poles (61.8522, -13.6129) (61.8522, -13.6853) (61.8446, -13.7082) (61.8236, -13.7082) knots 0 0 0 0 1 1 1 1
  spline S140 degree 3 poles (61.8236, -13.7082) (61.8008, -13.7082) (61.7951, -13.7405) (61.7951, -13.8777) knots 0 0 0 0 1 1 1 1
  spline S141 degree 3 poles (61.7951, -13.8777) (61.7951, -14.0644) (61.7741, -14.1444) (61.7227, -14.1596) knots 0 0 0 0 1 1 1 1
  spline S142 degree 3 poles (61.7227, -14.1596) (61.6808, -14.1692) (61.6503, -14.2397) (61.6331, -14.3635) knots 0 0 0 0 1 1 1 1
  spline S143 degree 3 poles (61.6331, -14.3635) (61.616, -14.4816) (61.6065, -14.5083) (61.5741, -14.5083) knots 0 0 0 0 1 1 1 1
  spline S144 degree 3 poles (61.5741, -14.5083) (61.5455, -14.5083) (61.5093, -14.3959) (61.5093, -14.3044) knots 0 0 0 0 1 1 1 1
  spline S145 degree 3 poles (61.5093, -14.3044) (61.5093, -14.272) (61.4998, -14.2377) (61.4903, -14.232) knots 0 0 0 0 1 1 1 1
  spline S146 degree 3 poles (61.4903, -14.232) (61.4788, -14.2263) (61.4712, -14.1996) (61.4712, -14.1749) knots 0 0 0 0 1 1 1 1
  spline S147 degree 3 poles (61.4712, -14.1749) (61.4712, -14.1406) (61.4636, -14.1311) (61.4426, -14.1406) knots 0 0 0 0 1 1 1 1
  spline S148 degree 3 poles (61.4426, -14.1406) (61.3836, -14.1615) (61.3588, -14.0892) (61.3569, -13.8968) knots 0 0 0 0 1 1 1 1
  spline S149 degree 3 poles (61.3569, -13.8968) (61.3569, -13.6872) (61.3588, -13.6891) (61.1702, -13.6891) knots 0 0 0 0 1 1 1 1
  line L69 (61.1702, -13.6891) -> (61.0712, -13.6891)
  line L70 (61.0712, -13.6891) -> (61.0712, -13.0319)
  spline S150 degree 3 poles (61.0712, -13.0319) (61.0712, -12.6699) (61.0674, -12.3747) (61.0616, -12.3747) knots 0 0 0 0 1 1 1 1
  spline S151 degree 3 poles (61.0616, -12.3747) (61.0559, -12.3747) (61.0293, -12.388) (61.0045, -12.4051) knots 0 0 0 0 1 1 1 1
  spline S152 degree 3 poles (61.0045, -12.4051) (60.9569, -12.4356) (60.9569, -12.4375) (60.9569, -12.7576) knots 0 0 0 0 1 1 1 1
  spline S153 degree 3 poles (60.9569, -12.7576) (60.9569, -12.9595) (60.9645, -13.0795) (60.9759, -13.0795) knots 0 0 0 0 1 1 1 1
  spline S154 degree 3 poles (60.9759, -13.0795) (60.9854, -13.0795) (60.995, -13.1176) (60.995, -13.1633) knots 0 0 0 0 1 1 1 1
  line L71 (60.995, -13.1633) -> (60.995, -13.2491)
  line L72 (60.995, -13.2491) -> (60.9035, -13.2548)
  spline S155 degree 3 poles (60.9035, -13.2548) (60.8407, -13.2586) (60.814, -13.2681) (60.8121, -13.2891) knots 0 0 0 0 1 1 1 1
  spline S156 degree 3 poles (60.8121, -13.2891) (60.8083, -13.3557) (60.8026, -13.3653) (60.7683, -13.3653) knots 0 0 0 0 1 1 1 1
  spline S157 degree 3 poles (60.7683, -13.3653) (60.7016, -13.3653) (60.6959, -13.4034) (60.7035, -13.7653) knots 0 0 0 0 1 1 1 1
  spline S158 degree 3 poles (60.7035, -13.7653) (60.7149, -14.2625) (60.7168, -14.5673) (60.713, -14.6226) knots 0 0 0 0 1 1 1 1
  spline S159 degree 3 poles (60.713, -14.6226) (60.7054, -14.6873) (60.734, -14.8245) (60.7759, -14.9235) knots 0 0 0 0 1 1 1 1
  spline S160 degree 3 poles (60.7759, -14.9235) (60.7987, -14.9788) (60.8045, -15.0264) (60.7968, -15.0759) knots 0 0 0 0 1 1 1 1
  spline S161 degree 3 poles (60.7968, -15.0759) (60.7778, -15.1788) (60.7778, -15.2169) (60.8045, -15.4798) knots 0 0 0 0 1 1 1 1
  spline S162 degree 3 poles (60.8045, -15.4798) (60.8197, -15.6455) (60.8349, -15.7217) (60.8559, -15.737) knots 0 0 0 0 1 1 1 1
  spline S163 degree 3 poles (60.8559, -15.737) (60.8845, -15.7579) (60.873, -15.8608) (60.8407, -15.8608) knots 0 0 0 0 1 1 1 1
  spline S164 degree 3 poles (60.8407, -15.8608) (60.8311, -15.8608) (60.8235, -15.8799) (60.8235, -15.9027) knots 0 0 0 0 1 1 1 1
  spline S165 degree 3 poles (60.8235, -15.9027) (60.8235, -15.9256) (60.8102, -15.9599) (60.7911, -15.9789) knots 0 0 0 0 1 1 1 1
  spline S166 degree 3 poles (60.7911, -15.9789) (60.7568, -16.0189) (60.7606, -16.017) (60.7206, -16.0018) knots 0 0 0 0 1 1 1 1
  spline S167 degree 3 poles (58.9852, -8.8275) (59.5376, -8.778) (60.1282, -8.5894) (60.5359, -8.3322) knots 0 0 0 0 1 1 1 1
  spline S168 degree 3 poles (60.5359, -8.3322) (61.155, -7.9455) (61.6712, -7.3474) (62.0084, -6.6254) knots 0 0 0 0 1 1 1 1
  spline S169 degree 3 poles (62.0084, -6.6254) (62.3304, -5.9377) (62.4828, -5.149) (62.4828, -4.1832) knots 0 0 0 0 1 1 1 1
  spline S170 degree 3 poles (62.4828, -4.1832) (62.4828, -2.8668) (62.2008, -1.9067) (61.5722, -1.1028) knots 0 0 0 0 1 1 1 1
  spline S171 degree 3 poles (61.5722, -1.1028) (60.8368, -0.1598) (59.7662, 0.3145) (58.4804, 0.2688) knots 0 0 0 0 1 1 1 1
  spline S172 degree 3 poles (58.4804, 0.2688) (57.8612, 0.246) (57.3964, 0.1393) (56.9278, -0.0874) knots 0 0 0 0 1 1 1 1
  spline S173 degree 3 poles (56.9278, -0.0874) (56.1639, -0.457) (55.5657, -1.1047) (55.3219, -1.8305) knots 0 0 0 0 1 1 1 1
  spline S174 degree 3 poles (55.3219, -1.8305) (55.2209, -2.1296) (55.1733, -2.3848) (55.1542, -2.7258) knots 0 0 0 0 1 1 1 1
  spline S175 degree 3 poles (55.1542, -2.7258) (55.1409, -2.9963) (55.1638, -3.1602) (55.2361, -3.303) knots 0 0 0 0 1 1 1 1
  spline S176 degree 3 poles (55.2361, -3.303) (55.3295, -3.4859) (55.4724, -3.5774) (55.7238, -3.6117) knots 0 0 0 0 1 1 1 1
  spline S177 degree 3 poles (55.7238, -3.6117) (55.9867, -3.6479) (56.2229, -3.585) (56.3639, -3.4402) knots 0 0 0 0 1 1 1 1
  spline S178 degree 3 poles (56.3639, -3.4402) (56.4858, -3.3145) (56.5201, -3.1964) (56.5392, -2.8401) knots 0 0 0 0 1 1 1 1
  spline S179 degree 3 poles (56.5392, -2.8401) (56.5696, -2.2477) (56.6344, -1.9905) (56.8306, -1.6895) knots 0 0 0 0 1 1 1 1
  spline S180 degree 3 poles (56.8306, -1.6895) (56.9125, -1.5657) (57.1126, -1.3542) (57.2421, -1.259) knots 0 0 0 0 1 1 1 1
  spline S181 degree 3 poles (57.2421, -1.259) (57.4212, -1.1256) (57.6803, -1.0075) (57.9374, -0.9428) knots 0 0 0 0 1 1 1 1
  spline S182 degree 3 poles (57.9374, -0.9428) (58.1337, -0.8932) (58.627, -0.8723) (58.8671, -0.9047) knots 0 0 0 0 1 1 1 1
  spline S183 degree 3 poles (58.8671, -0.9047) (59.3357, -0.9675) (59.7358, -1.158) (60.0691, -1.4781) knots 0 0 0 0 1 1 1 1
  spline S184 degree 3 poles (60.0691, -1.4781) (60.5473, -1.9391) (60.8388, -2.6211) (60.9473, -3.545) knots 0 0 0 0 1 1 1 1
  spline S185 degree 3 poles (60.9473, -3.545) (60.9892, -3.8898) (60.9892, -4.6975) (60.9473, -5.0499) knots 0 0 0 0 1 1 1 1
  spline S186 degree 3 poles (60.9473, -5.0499) (60.8445, -5.9396) (60.5568, -6.6292) (60.1015, -7.0788) knots 0 0 0 0 1 1 1 1
  spline S187 degree 3 poles (60.1015, -7.0788) (59.8272, -7.3512) (59.5586, -7.5036) (59.1719, -7.6064) knots 0 0 0 0 1 1 1 1
  spline S188 degree 3 poles (59.1719, -7.6064) (58.9985, -7.6522) (58.9566, -7.656) (58.5851, -7.6579) knots 0 0 0 0 1 1 1 1
  spline S189 degree 3 poles (58.5851, -7.6579) (58.2137, -7.6579) (58.1718, -7.6541) (58.0041, -7.6083) knots 0 0 0 0 1 1 1 1
  spline S190 degree 3 poles (58.0041, -7.6083) (57.2993, -7.4178) (56.823, -6.8997) (56.7278, -6.2196) knots 0 0 0 0 1 1 1 1
  spline S191 degree 3 poles (56.7278, -6.2196) (56.7163, -6.1415) (56.7106, -5.8767) (56.7125, -5.631) knots 0 0 0 0 1 1 1 1
  spline S192 degree 3 poles (56.7125, -5.631) (56.7182, -5.2347) (56.7144, -5.1699) (56.682, -5.0728) knots 0 0 0 0 1 1 1 1
  spline S193 degree 3 poles (56.682, -5.0728) (56.642, -4.949) (56.543, -4.8347) (56.4287, -4.7775) knots 0 0 0 0 1 1 1 1
  spline S194 degree 3 poles (56.4287, -4.7775) (56.261, -4.6918) (56.0058, -4.6746) (55.8096, -4.7356) knots 0 0 0 0 1 1 1 1
  spline S195 degree 3 poles (55.8096, -4.7356) (55.6476, -4.7851) (55.5486, -4.8728) (55.48, -5.0252) knots 0 0 0 0 1 1 1 1
  spline S196 degree 3 poles (55.48, -5.0252) (55.4324, -5.1299) (55.4247, -5.1738) (55.4171, -5.3738) knots 0 0 0 0 1 1 1 1
  spline S197 degree 3 poles (55.4171, -5.3738) (55.4133, -5.4995) (55.419, -5.6976) (55.4305, -5.8119) knots 0 0 0 0 1 1 1 1
  spline S198 degree 3 poles (55.4305, -5.8119) (55.5048, -6.5473) (55.5028, -6.7301) (55.4228, -7.5264) knots 0 0 0 0 1 1 1 1
  spline S199 degree 3 poles (55.4228, -7.5264) (55.4076, -7.6845) (55.3924, -7.9284) (55.3905, -8.0694) knots 0 0 0 0 1 1 1 1
  spline S200 degree 3 poles (55.3905, -8.0694) (55.3866, -8.4027) (55.419, -8.5132) (55.5562, -8.6523) knots 0 0 0 0 1 1 1 1
  spline S201 degree 3 poles (55.5562, -8.6523) (55.6781, -8.7742) (55.7829, -8.8123) (56.002, -8.8123) knots 0 0 0 0 1 1 1 1
  spline S202 degree 3 poles (56.002, -8.8123) (56.1372, -8.8123) (56.1848, -8.8028) (56.2706, -8.7628) knots 0 0 0 0 1 1 1 1
  spline S203 degree 3 poles (56.2706, -8.7628) (56.3868, -8.7094) (56.463, -8.6447) (56.522, -8.5494) knots 0 0 0 0 1 1 1 1
  spline S204 degree 3 poles (56.522, -8.5494) (56.5639, -8.4789) (56.6135, -8.3151) (56.6135, -8.237) knots 0 0 0 0 1 1 1 1
  spline S205 degree 3 poles (56.6135, -8.237) (56.6135, -8.2065) (56.6192, -8.1837) (56.6249, -8.1837) knots 0 0 0 0 1 1 1 1
  spline S206 degree 3 poles (56.6249, -8.1837) (56.6306, -8.1837) (56.6725, -8.2199) (56.7182, -8.2656) knots 0 0 0 0 1 1 1 1
  spline S207 degree 3 poles (56.7182, -8.2656) (56.8211, -8.3684) (57.1907, -8.557) (57.4707, -8.6485) knots 0 0 0 0 1 1 1 1
  spline S208 degree 3 poles (57.4707, -8.6485) (57.9851, -8.818) (58.4689, -8.8752) (58.9852, -8.8275) knots 0 0 0 0 1 1 1 1
  spline S209 degree 3 poles (73.0288, -8.6009) (73.3375, -8.5494) (73.5146, -8.3456) (73.5165, -8.0427) knots 0 0 0 0 1 1 1 1
  spline S210 degree 3 poles (73.5165, -8.0427) (73.5184, -7.8903) (73.4613, -7.7646) (73.3336, -7.635) knots 0 0 0 0 1 1 1 1
  spline S211 degree 3 poles (73.3336, -7.635) (73.1546, -7.454) (72.985, -7.4255) (72.5393, -7.4998) knots 0 0 0 0 1 1 1 1
  spline S212 degree 3 poles (72.5393, -7.4998) (72.343, -7.5341) (72.2878, -7.536) (72.2192, -7.5188) knots 0 0 0 0 1 1 1 1
  spline S213 degree 3 poles (72.2192, -7.5188) (72.0592, -7.475) (71.9506, -7.3016) (71.9106, -7.0254) knots 0 0 0 0 1 1 1 1
  spline S214 degree 3 poles (71.9106, -7.0254) (71.8992, -6.9473) (71.8916, -5.8634) (71.8935, -4.2784) knots 0 0 0 0 1 1 1 1
  spline S215 degree 3 poles (71.8935, -4.2784) (71.8935, -1.4971) (71.8935, -1.4819) (71.983, -1.2857) knots 0 0 0 0 1 1 1 1
  spline S216 degree 3 poles (71.983, -1.2857) (72.0783, -1.0742) (72.2154, -1.019) (72.5145, -1.0704) knots 0 0 0 0 1 1 1 1
  spline S217 degree 3 poles (72.5145, -1.0704) (72.6174, -1.0875) (72.7831, -1.1028) (72.8822, -1.1047) knots 0 0 0 0 1 1 1 1
  spline S218 degree 3 poles (72.8822, -1.1047) (73.0441, -1.1066) (73.0746, -1.1009) (73.1698, -1.0532) knots 0 0 0 0 1 1 1 1
  spline S219 degree 3 poles (73.1698, -1.0532) (73.3794, -0.9504) (73.5184, -0.7446) (73.5165, -0.5351) knots 0 0 0 0 1 1 1 1
  spline S220 degree 3 poles (73.5165, -0.5351) (73.5165, -0.3236) (73.4537, -0.1884) (73.3051, -0.0741) knots 0 0 0 0 1 1 1 1
  spline S221 degree 3 poles (73.3051, -0.0741) (73.1146, 0.0707) (72.8612, 0.0936) (72.3773, 0.0097) knots 0 0 0 0 1 1 1 1
  spline S222 degree 3 poles (72.3773, 0.0097) (71.9068, -0.0722) (71.5734, -0.1065) (71.2229, -0.1065) knots 0 0 0 0 1 1 1 1
  spline S223 degree 3 poles (71.2229, -0.1065) (70.8667, -0.1065) (70.6438, -0.0855) (70.1866, -0.0093) knots 0 0 0 0 1 1 1 1
  spline S224 degree 3 poles (70.1866, -0.0093) (69.7599, 0.0612) (69.5541, 0.0764) (69.3922, 0.0478) knots 0 0 0 0 1 1 1 1
  spline S225 degree 3 poles (69.3922, 0.0478) (69.1522, 0.0059) (69.0093, -0.0836) (68.9236, -0.2474) knots 0 0 0 0 1 1 1 1
  spline S226 degree 3 poles (68.9236, -0.2474) (68.8779, -0.3351) (68.8721, -0.3655) (68.8721, -0.5446) knots 0 0 0 0 1 1 1 1
  spline S227 degree 3 poles (68.8721, -0.5446) (68.8721, -0.7313) (68.8759, -0.7523) (68.9293, -0.8475) knots 0 0 0 0 1 1 1 1
  spline S228 degree 3 poles (68.9293, -0.8475) (69.0455, -1.0571) (69.2227, -1.1161) (69.6151, -1.0761) knots 0 0 0 0 1 1 1 1
  spline S229 degree 3 poles (69.6151, -1.0761) (70.0018, -1.038) (70.1332, -1.0418) (70.2247, -1.0932) knots 0 0 0 0 1 1 1 1
  spline S230 degree 3 poles (70.2247, -1.0932) (70.3123, -1.1428) (70.3733, -1.2285) (70.4304, -1.3809) knots 0 0 0 0 1 1 1 1
  spline S231 degree 3 poles (70.4304, -1.3809) (70.4704, -1.4857) (70.4723, -1.5181) (70.4781, -2.703) knots 0 0 0 0 1 1 1 1
  line L73 (70.4781, -2.703) -> (70.4838, -3.9165)
  line L74 (70.4838, -3.9165) -> (68.7102, -3.9165)
  line L75 (68.7102, -3.9165) -> (66.9348, -3.9165)
  line L76 (66.9348, -3.9165) -> (66.9424, -2.7125)
  spline S232 degree 3 poles (66.9424, -2.7125) (66.95, -1.5162) (66.95, -1.5047) (66.9938, -1.3733) knots 0 0 0 0 1 1 1 1
  spline S233 degree 3 poles (66.9938, -1.3733) (67.0281, -1.2723) (67.0567, -1.2209) (67.1195, -1.1618) knots 0 0 0 0 1 1 1 1
  spline S234 degree 3 poles (67.1195, -1.1618) (67.2357, -1.0475) (67.3481, -1.0361) (67.7672, -1.0875) knots 0 0 0 0 1 1 1 1
  spline S235 degree 3 poles (67.7672, -1.0875) (68.1006, -1.1294) (68.2568, -1.0952) (68.4111, -0.9466) knots 0 0 0 0 1 1 1 1
  spline S236 degree 3 poles (68.4111, -0.9466) (68.5559, -0.8094) (68.5902, -0.4551) (68.4816, -0.2398) knots 0 0 0 0 1 1 1 1
  spline S237 degree 3 poles (68.4816, -0.2398) (68.3578, 0.0002) (68.0892, 0.0936) (67.6548, 0.0478) knots 0 0 0 0 1 1 1 1
  spline S238 degree 3 poles (67.6548, 0.0478) (67.5272, 0.0345) (67.3881, 0.0155) (67.3443, 0.0059) knots 0 0 0 0 1 1 1 1
  spline S239 degree 3 poles (67.3443, 0.0059) (67.1253, -0.0398) (66.8338, -0.0722) (66.4642, -0.0874) knots 0 0 0 0 1 1 1 1
  spline S240 degree 3 poles (66.4642, -0.0874) (65.9251, -0.1103) (65.5517, -0.0874) (65.1669, -0.0074) knots 0 0 0 0 1 1 1 1
  spline S241 degree 3 poles (65.1669, -0.0074) (64.9307, 0.0402) (64.824, 0.0536) (64.6335, 0.0536) knots 0 0 0 0 1 1 1 1
  spline S242 degree 3 poles (64.6335, 0.0536) (64.3592, 0.0555) (64.2411, 0.0269) (64.0982, -0.0779) knots 0 0 0 0 1 1 1 1
  spline S243 degree 3 poles (64.0982, -0.0779) (63.8601, -0.2493) (63.8182, -0.7046) (64.0182, -0.9275) knots 0 0 0 0 1 1 1 1
  spline S244 degree 3 poles (64.0182, -0.9275) (64.1515, -1.0761) (64.3306, -1.118) (64.6545, -1.078) knots 0 0 0 0 1 1 1 1
  spline S245 degree 3 poles (64.6545, -1.078) (64.7631, -1.0647) (64.9288, -1.0513) (65.024, -1.0513) knots 0 0 0 0 1 1 1 1
  spline S246 degree 3 poles (65.024, -1.0513) (65.1726, -1.0494) (65.205, -1.0551) (65.2679, -1.0932) knots 0 0 0 0 1 1 1 1
  spline S247 degree 3 poles (65.2679, -1.0932) (65.3574, -1.1504) (65.4241, -1.2628) (65.4622, -1.4247) knots 0 0 0 0 1 1 1 1
  spline S248 degree 3 poles (65.4622, -1.4247) (65.4889, -1.539) (65.4908, -1.8743) (65.487, -4.3298) knots 0 0 0 0 1 1 1 1
  spline S249 degree 3 poles (65.487, -4.3298) (65.4812, -6.9759) (65.4793, -7.1111) (65.4469, -7.2007) knots 0 0 0 0 1 1 1 1
  spline S250 degree 3 poles (65.4469, -7.2007) (65.3936, -7.3378) (65.325, -7.4331) (65.2507, -7.4693) knots 0 0 0 0 1 1 1 1
  spline S251 degree 3 poles (65.2507, -7.4693) (65.1917, -7.4979) (65.1593, -7.4979) (64.9421, -7.475) knots 0 0 0 0 1 1 1 1
  spline S252 degree 3 poles (64.9421, -7.475) (64.8088, -7.4617) (64.6049, -7.4502) (64.4906, -7.4502) knots 0 0 0 0 1 1 1 1
  spline S253 degree 3 poles (64.4906, -7.4502) (64.3001, -7.4502) (64.2716, -7.4559) (64.1725, -7.5036) knots 0 0 0 0 1 1 1 1
  spline S254 degree 3 poles (64.1725, -7.5036) (64.0334, -7.5722) (63.9591, -7.6617) (63.9172, -7.8141) knots 0 0 0 0 1 1 1 1
  spline S255 degree 3 poles (63.9172, -7.8141) (63.8467, -8.0732) (63.9268, -8.3437) (64.1077, -8.4656) knots 0 0 0 0 1 1 1 1
  spline S256 degree 3 poles (64.1077, -8.4656) (64.1592, -8.4999) (64.2487, -8.5418) (64.3078, -8.5589) knots 0 0 0 0 1 1 1 1
  spline S257 degree 3 poles (64.3078, -8.5589) (64.4583, -8.6066) (64.8354, -8.6009) (65.1479, -8.5456) knots 0 0 0 0 1 1 1 1
  spline S258 degree 3 poles (65.1479, -8.5456) (65.7041, -8.4504) (66.6966, -8.4504) (67.2243, -8.5456) knots 0 0 0 0 1 1 1 1
  spline S259 degree 3 poles (67.2243, -8.5456) (67.5329, -8.6028) (67.9596, -8.6161) (68.1139, -8.578) knots 0 0 0 0 1 1 1 1
  spline S260 degree 3 poles (68.1139, -8.578) (68.4073, -8.5018) (68.5407, -8.3227) (68.5407, -8.0027) knots 0 0 0 0 1 1 1 1
  spline S261 degree 3 poles (68.5407, -8.0027) (68.5426, -7.7188) (68.434, -7.5417) (68.213, -7.4674) knots 0 0 0 0 1 1 1 1
  spline S262 degree 3 poles (68.213, -7.4674) (68.0835, -7.4236) (67.7825, -7.4236) (67.5996, -7.4674) knots 0 0 0 0 1 1 1 1
  spline S263 degree 3 poles (67.5996, -7.4674) (67.2891, -7.5398) (67.1405, -7.494) (67.0376, -7.2883) knots 0 0 0 0 1 1 1 1
  spline S264 degree 3 poles (67.0376, -7.2883) (66.95, -7.1111) (66.9386, -6.974) (66.9386, -5.9605) knots 0 0 0 0 1 1 1 1
  line L77 (66.9386, -5.9605) -> (66.9386, -5.0785)
  line L78 (66.9386, -5.0785) -> (68.7102, -5.0785)
  line L79 (68.7102, -5.0785) -> (70.4819, -5.0785)
  line L80 (70.4819, -5.0785) -> (70.4819, -5.77)
  spline S265 degree 3 poles (70.4819, -5.77) (70.48, -6.9626) (70.4495, -7.2521) (70.3085, -7.4121) knots 0 0 0 0 1 1 1 1
  spline S266 degree 3 poles (70.3085, -7.4121) (70.2056, -7.5283) (70.1523, -7.5321) (69.7313, -7.4655) knots 0 0 0 0 1 1 1 1
  spline S267 degree 3 poles (69.7313, -7.4655) (69.377, -7.4083) (69.156, -7.4636) (68.996, -7.6445) knots 0 0 0 0 1 1 1 1
  spline S268 degree 3 poles (68.996, -7.6445) (68.895, -7.7607) (68.855, -7.8979) (68.8683, -8.0789) knots 0 0 0 0 1 1 1 1
  spline S269 degree 3 poles (68.8683, -8.0789) (68.8874, -8.3227) (68.9998, -8.4789) (69.2227, -8.5685) knots 0 0 0 0 1 1 1 1
  spline S270 degree 3 poles (69.2227, -8.5685) (69.3198, -8.6066) (69.3598, -8.6104) (69.6627, -8.6104) knots 0 0 0 0 1 1 1 1
  spline S271 degree 3 poles (69.6627, -8.6104) (69.9332, -8.6085) (70.0723, -8.597) (70.4057, -8.5475) knots 0 0 0 0 1 1 1 1
  spline S272 degree 3 poles (70.4057, -8.5475) (70.6305, -8.5151) (70.9295, -8.4827) (71.0724, -8.477) knots 0 0 0 0 1 1 1 1
  spline S273 degree 3 poles (71.0724, -8.477) (71.3658, -8.4637) (71.882, -8.4942) (72.1202, -8.538) knots 0 0 0 0 1 1 1 1